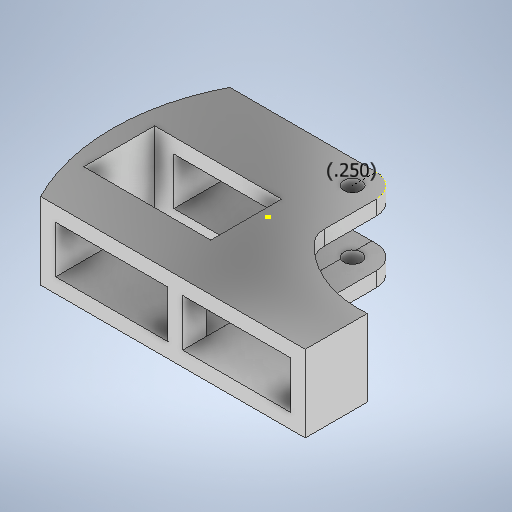
# Autodesk Inventor part: Part1
Saved by Autodesk Inventor 2025.1 (Build 291241000, 241)
## iProperties
Created: 2024-08-17
Part Number: Part1
Material: Generic
Document SubType Name: Modeling
Designer: vedan
Density: 1 g/cm^3
Appearance: Chrome - Polished
Author: vedan
Autodesk Inventor part; units mm, degrees
ref_plane "YZ Plane" through (0, 0, 0) normal (1, 0, 0) x (0, 1, 0)
ref_plane "XZ Plane" through (0, 0, 0) normal (0, 1, 0) x (-1, 0, 0)
sketch "Sketch1" plane through (0, 0, 0) normal (0, 1, 0) x (-1, 0, 0)
  line L0 (-35.5422, 25.4) -> (35.5422, 25.4)
  line L1 (35.5422, -25.4) -> (-10.1422, -25.4)
  line L2 (-35.5422, 8.7376) -> (-35.5422, 25.4)
  line L3 (-10.1422, -25.4) -> (-10.1422, -2.8194)
  arc A0 (-10.1422, -2.8194) -> (-35.5422, 8.7376) centre (-33.3502, -20.1353) ccw
  line L4 (35.5422, 25.4) -> (35.5422, -25.4) construction
  line L5 (35.5422, 0) -> (41.7398, 0) construction
  arc A1 (35.5422, -25.4) -> (35.5422, 25.4) centre (-13.4082, 0) ccw
  point P0 (0, 0)
  dimension "d2" = 22.5806
  dimension "d3" = 28.956
  dimension "d4" = 16.6624
  dimension "d5" = 50.8
  dimension "d7" = 71.0844
  dimension "d8" = 45.6844
  dimension "d12" = 6.1976
  constraints: 12 end point, 5 point on circle, 2 centre point, 2 horizontal, 2 vertical, 1 midpoint, 1 parallel
  measures "d2" distance of L1.end L3.end
  measures "d3" radius of A0
  measures "d4" distance of L2.start L0.start
  measures "d5" distance of L0.end L1.start
  measures "d7" distance of L0.start L0.end
  measures "d8" distance of L1.start L1.end
  measures "d12" distance of L5.start L5.end
extrude "Extrusion1" add sketch "Sketch1" along normal mid plane 20.6375
fillet "Fillet1" radius 6.35 2 edges at (10.1422, 0, -25.4) (10.1422, 0, -2.8194)
sketch "Sketch2" plane through (0, 10.3188, 0) normal (0, 1, 0) x (1, 0, 0)
  point P0 (0, 0)
sketch "Sketch3" plane through (0, 10.3188, 0) normal (0, 1, 0) x (1, 0, 0)
  line L0 (-36.6954, 6.35) -> (-2.5578, 6.35)
  line L1 (-2.5578, 6.35) -> (-2.5578, -12.7)
  line L2 (-2.5578, -12.7) -> (-36.6954, -12.7)
  line L3 (-36.6954, -12.7) -> (-36.6954, 6.35)
  line L4 (3.7922, 25.4) -> (-35.5422, 25.4) projected
  line L5 (35.5422, -25.4) -> (35.5422, -8.7376) projected
  point P0 (0, 0)
  dimension "d13" = 34.1376
  dimension "d14" = 19.05
  dimension "d15" = 19.05
  dimension "d16" = 38.1
  constraints: 8 end point, 2 parallel, 1 horizontal, 1 perpendicular
  measures "d13" distance of L0.start L0.end
  measures "d14" distance of L2.end L0.start
  measures "d15" distance from line of L4 L0.start
  measures "d16" distance between parallel lines of L5 L1
extrude "Extrusion2" cut sketch "Sketch3" against normal through all
sketch "Sketch4" plane through (-35.5422, 10.3188, 25.4) normal (0, 0, 1) x (1, 0, 0)
  line L0 (4.0132, -3.9751) -> (34.1884, -3.9751)
  line L1 (34.1884, -3.9751) -> (34.1884, -16.6751)
  line L2 (34.1884, -16.6751) -> (4.0132, -16.6751)
  line L3 (4.0132, -16.6751) -> (4.0132, -3.9751)
  line L4 (71.0844, -20.6375) -> (0, -20.6375) projected
  line L5 (0, 0) -> (0, -20.6375) projected
  line L6 (38.1508, -3.9624) -> (67.1322, -3.9624)
  line L7 (67.1322, -3.9624) -> (67.1322, -16.6624)
  line L8 (67.1322, -16.6624) -> (38.1508, -16.6624)
  line L9 (38.1508, -16.6624) -> (38.1508, -3.9624)
  line L10 (0, 0) -> (71.0844, 0) projected
  point P0 (35.5422, -10.3188)
  point P1 (34.1884, -10.3251)
  dimension "d19" = 30.1752
  dimension "d20" = 3.9624
  dimension "d21" = 12.7
  dimension "d22" = 4.0132
  dimension "d23" = 3.9624
  dimension "d24" = 28.9814
  dimension "d25" = 3.9624
  dimension "d26" = 12.7
  constraints: 16 end point, 4 parallel, 2 horizontal, 2 perpendicular, 1 midpoint
  measures "d19" distance of L0.start L0.end
  measures "d20" distance between parallel lines of L2 L4
  measures "d21" distance of L2.end L0.start
  measures "d22" distance between parallel lines of L5 L3
  measures "d23" distance from line of point (34.188, -10.325) L9
  measures "d24" distance of L6.start L6.end
  measures "d25" distance between parallel lines of L10 L6
  measures "d26" distance of L6.end L7.end
extrude "Extrusion3" cut sketch "Sketch4" against normal through all
sketch "Sketch5" plane through (-35.5422, -10.3188, -25.4) normal (0, 0, -1) x (-1, 0, 0)
  line L0 (-38.1508, 16.6751) -> (-34.1884, 16.6751)
  line L1 (-34.1884, 16.6751) -> (-34.1884, 3.9624)
  line L2 (-34.1884, 3.9624) -> (-38.1508, 3.9624)
  line L3 (-38.1508, 3.9624) -> (-38.1508, 16.6751)
  point P0 (-35.5422, 10.3188)
  constraints: 8 end point, 2 parallel, 1 horizontal, 1 perpendicular
ref_plane "Work Plane1" through (-35.5422, 10.3188, 19.05) normal (0, 0, 1) x (1, 0, 0)
extrude "Extrusion4" cut sketch "Sketch5" against normal up to surface (44.45 mm away)
sketch "Sketch6" plane through (0, 10.3188, 0) normal (0, 1, 0) x (1, 0, 0)
  arc A0 (10.1422, 19.05) -> (3.7922, 25.4) centre (3.7922, 19.05) ccw projected
  point P0 (0, 0)
  constraints: 1 coincident
hole "Hole1" at (3.7922, 10.3188, -19.05) direction (0, -1, 0) diameter 4.7625 end through all
sketch "Sketch7" plane through (0, 10.3188, 0) normal (0, 1, 0) x (1, 0, 0)
  arc A0 (10.1422, 19.05) -> (3.7922, 25.4) centre (3.7922, 19.05) ccw construction
  line L0 (3.7922, 19.05) -> (3.7922, 25.4) construction
  point P0 (0, 0)
  dimension "d39" = 6.35
  constraints: 2 end point, 1 vertical
  measures "d39" distance of L0.start L0.end
body "Solid1"
